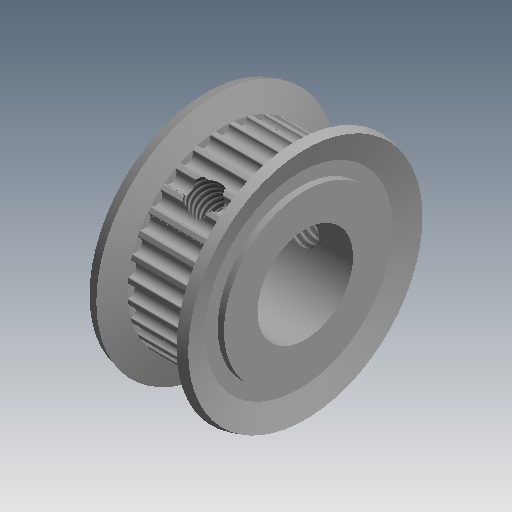
# Autodesk Inventor part: GPA32GT2060-A-P10_b
Saved by Autodesk Inventor 2020 (Build 240168000, 168)
## iProperties
Part Number: GPA32GT2060-A-P10_b
Material: Generic
Catalog Web Link: www.cadenas.de
Description: GPA__GT2040, GPA__GT2060, GPA__GT2090_body-High Torque Timing Pulleys 2GT Type
Vendor: MISUMI
Document SubType Name: Modeling
Designer: partserver
Manufacturer: MISUMI
Mass: 2.37112 g
Surface Area: 24.3062 cm^2
Volume: 2.37112 cm^3
Density: 1 g/cm^3
Appearance: PSOLRGB-192-192-192
Category: PARTsolutions
Company: MISUMI
PSOL_IDENT_0: {$CADENAS_DATA\23d-libs\misumi\metric\51_timing_pulleys\gpa__gt2\gpa_gt2.prj},385 {VTYP=3D},{NB=GPA3
PSOL_IDENT_1: 2GT2060-A-P10_b},{LINA=GPA32GT2060-A-P10},{NN=GPA__GT2040, GPA__GT2060, GPA__GT2090_body},{DATE=17.0
PSOL_IDENT_2: 1.2019 09:47:54},{GEOMDATE=17.12.2018 08:21:00},{VERSION=},{LINEID=120},{WBVAR=TNW,PS,SBS,DD,Z,J,Q,R
PSOL_IDENT_3: ,S,T,ALT1,ALT2,M,QSC,QFC,QTC,ALT3,K,KSC,KFC,KTC,ALT4,ZM,ZSC,ZFC,ZTC,ALT5,BC,ALT6,ALT7,ALT8,FC},{WBNU
PSOL_IDENT_4: MERIC=DD,Z,J,Q,R,S,T,QSC,QFC,QTC,K,KSC,KFC,KTC,ZSC,ZFC,ZTC,BC,FC}  {NB=GPA32GT2060-A-P10_b},{LINA=GP
PSOL_IDENT_5: A32GT2060-A-P10},{KT=DUMMY},{PN=GPA32GT2060-A-P10},{TYPE=GPA},{NT=32},{TNW=GT2060},{BW=6},{A=7.0},{W=
PSOL_IDENT_6: 10.3},{L=18.0},{PS=A},{PSA= 'A','B' },{SBS=P},{SBSALG= 'H','Round Hole','P','Round Hole+Tap','V','St
PSOL_IDENT_7: epped Hole','Y','Both Ends Stepped Hole' },{DD=10.00},{DDALG=[5:6/1],[6.35],[7:10/1]},{DDHA=[5:6/1],
PSOL_IDENT_8: [6.35],[7:13/1]},{DDHB=[5:6/1],[6.35],[7:9/1]},{DDPA=[5:6/1],[6.35],[7:10/1]},{DDPB=[5:6/1]},{DDNA=}
PSOL_IDENT_9: ,{DDNB=},{DDNKA=0},{DDNKB=0},{DDVA=[5:6/1],[6.35],[7:11/1]},{DDVFB=[5:6/1],[6.35],[7:7/1]},{DDYA=[5:
PSOL_IDENT_10: 11/1]},{Z=0},{ZALG=0},{ZMIN=12},{ZAMAX=13},{ZBMAX=9},{J=0.0},{JALG=0},{JMAX=8.3},{Q=0},{R=0},{QRALG=
PSOL_IDENT_11: 0},{QRMIN=12},{QRMAX=13},{S=0.0},{SALG=0},{SMAX=4.300},{T=0.0},{TALG=0},{TMAX=5.000},{PD=20.37},{OD=
PSOL_IDENT_12: 19.86},{D=13},{DE=17},{DDZ=10},{F=25},{E=17},{BB=0},{TT=0},{M1=4},{AC=M4x3},{ALT1=},{ALT1A= '','w/o
PSOL_IDENT_13: Set Screw Angle','-KC90','with KC90 (Set Screw Angle)' },{ANG=123.75},{ALT2=},{ALT2A= '','Not applic
PSOL_IDENT_14: able' },{M=N/A},{MALG= 'N/A' },{MM=0.000},{MPHD=0.000},{MA= 'N/A' },{MSA= 'N/A' },{QSC=0.0},{QSCA=0}
PSOL_IDENT_15: ,{QFC=0.0},{QFCA=0},{QTC=0.0},{QTCA=0},{QPCDMIN=14},{QPCDMINALG=14},{QPCDMAX=13},{ALT2PN=},{ALT3=},{
PSOL_IDENT_16: ALT3A= '','Not applicable' },{K=0.0},{KA=0},{KAMIN=4},{KAMAX=0},{KSMAX=0},{KSC=0.0},{KSCA=0},{KFC=0.
PSOL_IDENT_17: 0},{KFCA=0},{KTC=0.0},{KTCA=0},{KSCMIN=14.000},{KPCDMIN=14.000},{KPCDMINALG=18.000},{KPCDMAX=13.000}
PSOL_IDENT_18: ,{ALT3PN=},{ALT4=},{ALT4ALG= '','Not applicable' },{ALT4MIN=20.500},{ALT4MAX=6.500},{ZM=N/A},{ZMALG=
PSOL_IDENT_19: 'N/A' },{ZMFTALG= 'N/A' },{ZMSALG= 'N/A' },{ZMDD1=0.0},{ZMDD2=0.0},{ZMHH=0.0},{ZSC=0.0},{ZSCALG=[0]
PSOL_IDENT_20: },{ZFC=0.0},{ZFCALG=[0]},{ZTC=0.0},{ZTCALG=[0]},{ZPCDMIN=0.000},{ZPCDMINALG=0.000},{ZPCDMAX=13.000},
PSOL_IDENT_21: {ALT4PN=},{ALT5=},{ALT5ALG= '','Not applicable' },{ALT5PN=},{BC=0.0},{BCALG=0},{BCMIN=7.000},{BCMAX=
PSOL_IDENT_22: 7.700},{ALT6=},{ALT7=},{ALT7ALG= '','w/o Flange Attached on One Side Only','-RFC','with RFC (Flange
PSOL_IDENT_23: Attached on The Boss Side Only)','-LFC','with LFC (Flange Attached on The Opposite Side Only)' },{AL
PSOL_IDENT_24: T8=},{ALT8ALG='','w/o FC (Flange Cut)','-FC','with FC (Flange Cut)'},{ALT8PN=},{FC=0.0},{FCA=0},{ODA
PSOL_IDENT_25: INT=23.000},{FCMIN=21},{FCMAX=23},{WLBC=10.3},{SL=5},{SL2=5},{KTT=5},{KYY=4.93},{TAP=0}
NB: GPA32GT2060-A-P10_b
NN: GPA__GT2040, GPA__GT2060, GPA__GT2090_body
NT: 32
NBSYN: $PN._b
LINA: GPA32GT2060-A-P10
CATALOG: Misumi
PN: GPA32GT2060-A-P10
TNW: GT2060
A: 7
W: 10.3
L: 18
PS: A
SBS: Round Hole+Tap
DD: 10
Z: 0
J: 0
Q: 0
R: 0
S: 0
T: 0
PD: 20.37
OD: 19.86
D: 13
F: 25
E: 17
AC: M4x3
ALT1: w/o Set Screw Angle
ALT2: Not applicable
M: N/A
QSC: 0
QFC: 0
QTC: 0
ALT3: Not applicable
K: 0
KSC: 0
KFC: 0
KTC: 0
ALT4: Not applicable
ZM: N/A
ZMDD1: 0
ZMDD2: 0
ZMHH: 0
ZSC: 0
ZFC: 0
ZTC: 0
ALT5: Not applicable
BC: 0
ALT6: w/o Flange not Attached
ALT7: w/o Flange Attached on One Side Only
ALT8: w/o FC (Flange Cut)
FC: 0
SUPPLIER: MISUMI
ARTICLENO: GPA32GT2060-A-P10_b
BOMINFO: GPA32GT2060-A-P10
CREATOR: CADENAS GmbH
Title: GPA32GT2060-A-P10
Author: Cadenas PARTsolutions
Comments: High Torque Timing Pulleys 2GT Type
Autodesk Inventor part; units mm, degrees
ref_plane "YZ Plane" through (0, 0, 0) normal (1, 0, 0) x (0, 1, 0)
ref_plane "XZ Plane" through (0, 0, 0) normal (0, 1, 0) x (-1, 0, 0)
ref_plane "XY Plane" through (0, 0, 0) normal (0, 0, 1) x (1, 0, 0)
sketch "Sketch_16" plane through (0, 0, 0) normal (0, 0, 1) x (1, 0, 0)
  line L0 (5.15, 0) -> (-5.15, 0)
  line L1 (-5.15, 0) -> (-5.15, 8.5)
  line L2 (-5.15, 8.5) -> (-3.5, 8.5)
  line L3 (-3.5, 8.5) -> (-3.5, 9.93)
  line L4 (-3.5, 9.93) -> (3.5, 9.93)
  line L5 (3.5, 9.93) -> (3.5, 8.5)
  line L6 (3.5, 8.5) -> (5.15, 8.5)
  line L7 (5.15, 8.5) -> (5.15, 0)
  line L8 (5.15, 0) -> (-5.15, 0)
  constraints: 18 end point
revolve "Revolution1" add sketch "Sketch_16" angle 360 about axis through (5.15, 0, 0) along (1, 0, 0)
sketch "Sketch_18" plane through (0, 0, 0) normal (1, 0, 0) x (0, 1, 0)
  line L0 (10.1405, 0.9509) -> (9.8885, 0.9273)
  line L1 (9.8885, 0.9273) -> (9.8993, 0.793)
  arc A0 (9.7974, 0.6724) -> (9.8993, 0.793) centre (9.7876, 0.784) ccw
  arc A1 (9.7974, 0.6724) -> (9.7974, -0.6724) centre (9.856, 0) ccw
  arc A2 (9.8993, -0.793) -> (9.7974, -0.6724) centre (9.7876, -0.784) ccw
  line L2 (9.8993, -0.793) -> (9.8885, -0.9273)
  line L3 (9.8885, -0.9273) -> (10.1405, -0.9509)
  arc A3 (10.1405, -0.9509) -> (10.1405, 0.9509) centre (0, 0) ccw
  constraints: 8 end point, 8 point on circle, 4 centre point
extrude "Extrusion1" cut sketch "Sketch_18" along normal mid plane 7
pattern_circular "Circular Pattern1" count 32 over 360 about axis through (0, 0, 0) along (1, 0, 0) of "Extrusion1"
sketch "Sketch_20" plane through (0, 0, 0) normal (0, 0, 1) x (1, 0, 0)
  line L0 (50, 0) -> (-50, 0)
  line L1 (3.5, 9.93) -> (3.5, 8.5)
  line L2 (3.5, 8.5) -> (4.5, 8.5)
  line L3 (4.5, 8.5) -> (4.5, 9.7983)
  line L4 (4.5, 9.7983) -> (5.1546, 12.2412)
  line L5 (5.1546, 12.2412) -> (4.1886, 12.5)
  line L6 (4.1886, 12.5) -> (3.5, 9.93)
  constraints: 14 end point
revolve "Revolution2" add sketch "Sketch_20" angle 360 about axis through (50, 0, 0) along (1, 0, 0)
sketch "Sketch_21" plane through (0, 0, 0) normal (0, 0, 1) x (1, 0, 0)
  line L0 (50, 0) -> (-50, 0)
  line L1 (-5.1546, 12.2412) -> (-4.5, 9.7983)
  line L2 (-4.5, 9.7983) -> (-4.5, 8.5)
  line L3 (-4.5, 8.5) -> (-3.5, 8.5)
  line L4 (-3.5, 8.5) -> (-3.5, 9.93)
  line L5 (-3.5, 9.93) -> (-4.1886, 12.5)
  line L6 (-4.1886, 12.5) -> (-5.1546, 12.2412)
  constraints: 14 end point
revolve "Revolution3" add sketch "Sketch_21" angle 360 about axis through (50, 0, 0) along (1, 0, 0)
sketch "Sketch5" plane through (5.15, 0, 0) normal (1, 0, 0) x (0, 0, -1)
  point P0 (0, 0)
hole "Hole1" at (5.15, 0, 0) direction (-1, 0, 0) diameter 10 depth 10.3
sketch "Sketch_23" plane through (0, 0, 0) normal (1, 0, 0) x (0, 0, -1)
  line L0 (0, 0) -> (0, 9.93)
  line L1 (0, 9.93) -> (1.621, 9.93)
  line L2 (1.621, 9.93) -> (1.621, 0)
  line L3 (1.621, 0) -> (0, 0)
  line L4 (0, 0) -> (0, 9.93)
  constraints: 10 end point
revolve "Revolution4" cut sketch "Sketch_23" angle 360 about axis through (0, 0, 0) along (0, -1, 0)
thread "Thread1" size "M4x0.7" class "6H" standard "ISO Metric profile" length 4.93
sketch "Sketch_24" plane through (0, 0, 0) normal (1, 0, 0) x (0, 0, -1)
  line L0 (0, 0) -> (8.2565, -5.5168)
  line L1 (8.2565, -5.5168) -> (7.3559, -6.8646)
  line L2 (7.3559, -6.8646) -> (-0.9006, -1.3478)
  line L3 (-0.9006, -1.3478) -> (0, 0)
  line L4 (0, 0) -> (8.2565, -5.5168)
  constraints: 10 end point
revolve "Revolution5" cut sketch "Sketch_24" angle 360 about axis through (0, 0, 0) along (0, 0.5555702, 0.8314696)
thread "Thread2" size "M4x0.7" class "6H" standard "ISO Metric profile" length 4.93
ref_plane "to_Screw_A1_XY" through (0, 5, 0) normal (0, 1, 0) x (1, 0, 0)
ref_plane "to_Screw_A1_YZ" through (0, 5, 0) normal (1, 0, 0) x (0, 0, -1)
ref_plane "to_Screw_A1_ZX" through (0, 5, 0) normal (0, 0, -1) x (0, 1, 0)
ref_plane "to_Screw_A2_XY" through (0, -2.7779, -4.1573) normal (0, -0.5555702, -0.8314696) x (1, 0, 0)
ref_plane "to_Screw_A2_YZ" through (0, -2.7779, -4.1573) normal (1, 0, 0) x (0, -0.8314696, 0.5555702)
ref_plane "to_Screw_A2_ZX" through (0, -2.7779, -4.1573) normal (0, -0.8314696, 0.5555702) x (0, -0.5555702, -0.8314696)
body "Solid1"
